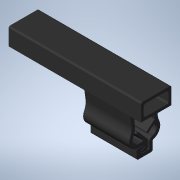
# Autodesk Inventor part: 1247168 ASCF-M-23-S DM 2.1-3.4
Saved by Autodesk Inventor 2021 (Build 250183000, 183)
## iProperties
Created: 2026-04-08
Part Number: 1247168 ASCF-M-23-S DM 2.1-3.4
Material: Generic
Catalog Web Link: www.3dfindit.com
Description: ASCF-M-inscription label holder
Vendor: FESTO
Document SubType Name: Modeling
Designer: psAdmin
Manufacturer: FESTO
Mass: 0.293788 g
Surface Area: 11.3078 cm^2
Volume: 0.293788 cm^3
Density: 1 g/cm^3
Appearance: PSOLRGB-176-176-176
Category: PARTsolutions
Company: FESTO
Title: 1247168 ASCF-M-23-S DM 2.1-3.4
Author: Cadenas PARTsolutions
Comments: inscription label holder
PSOL_IDENT_0: {$CADENAS_DATA/23d-libs/festo/parts/a/ascf/ascf_m.prj},201 {VTYP=3D},{NB=1247168 ASCF-M-23-S DM 2.1-
PSOL_IDENT_1: 3.4},{LINA=1247168 ASCF-M-23-S DM 2.1-3.4},{NN=ASCF-M},{DATE=10.03.2026 09:30:44},{GEOMDATE=01.09.20
PSOL_IDENT_2: 15 13:26:34},{VERSION=},{LINEID=120},{WBVAR=},{WBNUMERIC=}  {NB=1247168 ASCF-M-23-S DM 2.1-3.4},{LIN
PSOL_IDENT_3: A=1247168 ASCF-M-23-S DM 2.1-3.4},{KT=DUMMY},{TNR=1247168},{TYP=ASCF-M-23-S DM 2.1-3.4},{H=10.3},{KA
PSOL_IDENT_4: BEL=2.1-3.4},{KMIN=2.1},{KMAX=3.4},{VERS=3}
NB: 1247168 ASCF-M-23-S DM 2.1-3.4
NN: ASCF-M
NT: inscription label holder
NBSYN: $TNR. $TYP.
LINA: 1247168 ASCF-M-23-S DM 2.1-3.4
CATALOG: Festo
TNR: 1247168
TYP: ASCF-M-23-S DM 2.1-3.4
H: 10.3
KABEL: 2.1-3.4
SUPPLIER: FESTO
ARTICLENO: 1247168 ASCF-M-23-S DM 2.1-3.4
BOMINFO: 1247168 ASCF-M-23-S DM 2.1-3.4
CREATOR: CADENAS GmbH
Autodesk Inventor part; units mm, degrees
sketch "Sketch_11" plane through (0, 0, 0) normal (1, 0, 0) x (0, 1, 0)
  arc A0 (-1.1346, 2.5361) -> (-3.3951, 1.4765) centre (-1.84, 1.1) ccw
  arc A1 (-3.4923, 1.4) -> (-3.3951, 1.4765) centre (-3.4923, 1.5) ccw
  line L0 (-3.4923, 1.4) -> (-4.84, 1.4)
  arc A2 (-4.84, 1.4) -> (-5.14, 1.1) centre (-4.84, 1.1) ccw
  line L1 (-5.14, 1.1) -> (-5.14, -1.1)
  arc A3 (-5.14, -1.1) -> (-4.84, -1.4) centre (-4.84, -1.1) ccw
  line L2 (-4.84, -1.4) -> (-3.4923, -1.4)
  arc A4 (-3.3951, -1.4765) -> (-3.4923, -1.4) centre (-3.4923, -1.5) ccw
  arc A5 (-3.3951, -1.4765) -> (-1.1346, -2.5361) centre (-1.84, -1.1) ccw
  arc A6 (0.4796, -2.2735) -> (-1.1346, -2.5361) centre (0.1042, -5.0583) ccw
  line L3 (0.4796, -2.2735) -> (2.16, -2.5)
  line L4 (2.16, -2.5) -> (2.16, 2.5)
  line L5 (2.16, 2.5) -> (0.4796, 2.2735)
  arc A7 (-1.1346, 2.5361) -> (0.4796, 2.2735) centre (0.1042, 5.0583) ccw
  circle A8 centre (0, 0) radius 1.45
  constraints: 16 point on circle, 12 end point, 9 centre point
extrude "Extrusion1" add sketch "Sketch_11" against normal blind 8
sketch "Sketch_12" plane through (2, 0, 0) normal (1, 0, 0) x (0, 0, -1)
  line L0 (-2.65, 4.86) -> (-2.65, 2.16)
  line L1 (-2.65, 2.16) -> (2.65, 2.16)
  line L2 (2.65, 2.16) -> (2.65, 4.86)
  arc A0 (2.65, 4.86) -> (2.35, 5.16) centre (2.35, 4.86) ccw
  line L3 (2.35, 5.16) -> (-2.35, 5.16)
  arc A1 (-2.35, 5.16) -> (-2.65, 4.86) centre (-2.35, 4.86) ccw
  constraints: 8 end point, 4 point on circle, 2 centre point
extrude "Extrusion2" add sketch "Sketch_12" against normal blind 23
sketch "Sketch_13" plane through (2, 0, 0) normal (1, 0, 0) x (0, 0, -1)
  arc A0 (-2.15, 2.96) -> (-1.85, 2.66) centre (-1.85, 2.96) ccw
  line L0 (-1.85, 2.66) -> (1.85, 2.66)
  arc A1 (1.85, 2.66) -> (2.15, 2.96) centre (1.85, 2.96) ccw
  line L1 (2.15, 2.96) -> (2.15, 4.36)
  arc A2 (2.15, 4.36) -> (1.85, 4.66) centre (1.85, 4.36) ccw
  line L2 (1.85, 4.66) -> (-1.85, 4.66)
  arc A3 (-1.85, 4.66) -> (-2.15, 4.36) centre (-1.85, 4.36) ccw
  line L3 (-2.15, 4.36) -> (-2.15, 2.96)
  constraints: 8 end point, 8 point on circle, 4 centre point
extrude "Extrusion3" cut sketch "Sketch_13" against normal blind 23
sketch "Sketch_14" plane through (0, 0, 0) normal (1, 0, 0) x (0, 1, 0)
  arc A0 (-1.4233, 2.0091) -> (-2.84, 1.1) centre (-1.84, 1.1) ccw
  line L0 (-2.84, 1.1) -> (-2.84, 0.5446)
  arc A1 (-2.84, 0.5446) -> (-2.5075, 0.3948) centre (-2.64, 0.5446) ccw
  line L1 (-2.5075, 0.3948) -> (-1.3404, 1.4271)
  arc A2 (-1.0422, 1.09) -> (-1.3404, 1.4271) centre (-1.1913, 1.2585) ccw
  line L2 (-1.0422, 1.09) -> (-2.84, -0.5)
  line L3 (-2.84, -0.5) -> (-4.24, -0.5)
  arc A3 (-4.44, -0.3) -> (-4.24, -0.5) centre (-4.24, -0.3) ccw
  line L4 (-4.44, -0.3) -> (-4.44, 0.35)
  arc A4 (-4.24, 0.55) -> (-4.44, 0.35) centre (-4.24, 0.35) ccw
  arc A5 (-4.04, 0.35) -> (-4.24, 0.55) centre (-4.24, 0.35) ccw
  line L5 (-4.04, 0.35) -> (-4.04, 0.3)
  arc A6 (-4.04, 0.3) -> (-3.74, 0) centre (-3.74, 0.3) ccw
  arc A7 (-3.74, 0) -> (-3.44, 0.3) centre (-3.74, 0.3) ccw
  line L6 (-3.44, 0.3) -> (-3.44, 1.1)
  arc A8 (-3.1629, 2) -> (-3.44, 1.1) centre (-1.84, 1.1) ccw
  line L7 (-3.1629, 2) -> (-3.54, 2)
  line L8 (-3.54, 2) -> (-3.54, 0.3)
  arc A9 (-3.74, 0.1) -> (-3.54, 0.3) centre (-3.74, 0.3) ccw
  arc A10 (-3.94, 0.3) -> (-3.74, 0.1) centre (-3.74, 0.3) ccw
  line L9 (-3.94, 0.3) -> (-3.94, 0.4)
  arc A11 (-3.94, 0.4) -> (-4.14, 0.6) centre (-4.14, 0.4) ccw
  line L10 (-4.14, 0.6) -> (-4.34, 0.6)
  arc A12 (-4.34, 0.6) -> (-4.54, 0.4) centre (-4.34, 0.4) ccw
  line L11 (-4.54, 0.4) -> (-4.54, -0.6)
  arc A13 (-4.54, -0.6) -> (-4.34, -0.8) centre (-4.34, -0.6) ccw
  line L12 (-4.34, -0.8) -> (-3.4923, -0.8)
  arc A14 (-2.8119, -1.3353) -> (-3.4923, -0.8) centre (-3.4923, -1.5) ccw
  arc A15 (-2.8119, -1.3353) -> (-1.4233, -2.0091) centre (-1.84, -1.1) ccw
  arc A16 (-0.9842, -1.8433) -> (-1.4233, -2.0091) centre (-0.0025, -5.109) ccw
  line L13 (-0.9842, -1.8433) -> (-1.95, -0.6923)
  arc A17 (-1.6053, -0.403) -> (-1.95, -0.6923) centre (-1.7776, -0.5477) ccw
  line L14 (-1.6053, -0.403) -> (-0.4886, -1.7338)
  arc A18 (0.34, -1.7162) -> (-0.4886, -1.7338) centre (-0.0025, -5.109) ccw
  line L15 (0.34, -1.7162) -> (2.16, -1.9)
  line L16 (2.16, -1.9) -> (2.16, 1.9)
  line L17 (2.16, 1.9) -> (0.34, 1.7162)
  arc A19 (-1.4233, 2.0091) -> (0.34, 1.7162) centre (-0.0025, 5.109) ccw
  constraints: 40 point on circle, 36 end point, 20 centre point
extrude "Extrusion4" cut sketch "Sketch_14" against normal blind 8
sketch "Sketch_4" plane through (0, 0, 0) normal (1, 0, 0) x (0, 1, 0)
  line L0 (2.2363, -0.1854) -> (0.8628, -1.3489)
  line L1 (0.8628, -1.3489) -> (1.186, -1.7304)
  line L2 (1.186, -1.7304) -> (2.5595, -0.5669)
  line L3 (2.5595, -0.5669) -> (2.2363, -0.1854)
  constraints: 8 end point
extrude "Extrusion5" add sketch "Sketch_4" against normal blind 8
sketch "Sketch_5" plane through (0, 0, 0) normal (1, 0, 0) x (0, 1, 0)
  line L0 (1.186, 1.7304) -> (0.8628, 1.3489)
  line L1 (0.8628, 1.3489) -> (2.2363, 0.1854)
  line L2 (2.2363, 0.1854) -> (2.5595, 0.5669)
  line L3 (2.5595, 0.5669) -> (1.186, 1.7304)
  constraints: 8 end point
extrude "Extrusion6" add sketch "Sketch_5" against normal blind 8
ref_plane "CP_XY" through (2, 5.16, 0) normal (1, 0, 0) x (0, 0, -1)
ref_plane "CP_YZ" through (2, 5.16, 0) normal (0, 0, -1) x (0, 1, 0)
ref_plane "CP_ZX" through (2, 5.16, 0) normal (0, 1, 0) x (1, 0, 0)
ref_plane "KTN_XY" through (0, 0, 0) normal (1, 0, 0) x (0, 0, -1)
ref_plane "KTN_YZ" through (0, 0, 0) normal (0, 0, -1) x (0, 1, 0)
ref_plane "KTN_ZX" through (0, 0, 0) normal (0, 1, 0) x (1, 0, 0)
body "Solid1"
